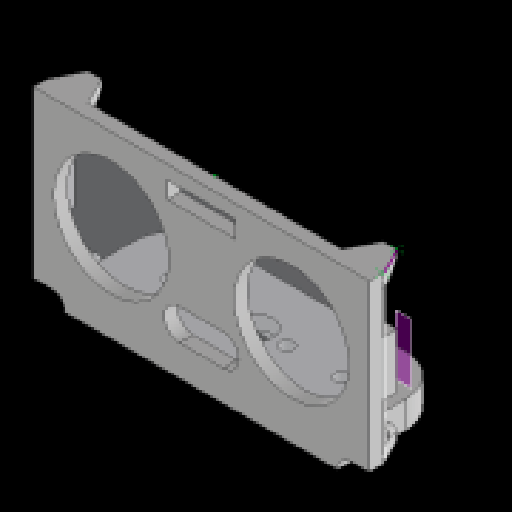
# Autodesk Inventor part: ultrasomicHolder
Saved by Autodesk Inventor 2024.3 (Build 283343010, 343A)
## iProperties
Created: 2025-05-13
Part Number: ultrasomicHolder
Material: Generic
Document SubType Name: Modeling
Designer: Oleg Kelner
Density: 1 g/cm^3
Appearance: Default
Author: Oleg Kelner
Autodesk Inventor part; units mm, degrees
ref_plane "YZ Plane" through (0, 0, 0) normal (1, 0, 0) x (0, 1, 0)
ref_plane "XZ Plane" through (0, 0, 0) normal (0, 1, 0) x (-1, 0, 0)
ref_plane "XY Plane" through (0, 0, 0) normal (0, 0, 1) x (1, 0, 0)
ref_plane "Work Plane1" through (0, 0, 0) normal (0, 0, 1) x (1, 0, 0)
sketch "Sketch1" plane through (0, 0, 0) normal (0, 0, 1) x (1, 0, 0)
  line L0 (-22.65, -10.15) -> (22.65, -10.15) construction
  line L1 (22.65, -10.15) -> (22.65, 10.15) construction
  line L2 (22.65, 10.15) -> (-22.65, 10.15) construction
  line L3 (-22.65, 10.15) -> (-22.65, -10.15) construction
  line L4 (3.2, -5.55) -> (-3.2, -5.55) construction
  arc A0 (3.2, -9.15) -> (3.2, -5.55) centre (3.2, -7.35) ccw construction
  line L5 (-3.2, -9.15) -> (3.2, -9.15) construction
  arc A1 (-3.2, -5.55) -> (-3.2, -9.15) centre (-3.2, -7.35) ccw construction
  circle A2 centre (-13.25, 0) radius 7.95 construction
  circle A3 centre (13.25, 0) radius 7.95 construction
  circle A4 centre (-21.75, -9.25) radius 0.75 construction
  circle A5 centre (-21.75, 9.25) radius 0.75 construction
  circle A6 centre (21.75, 9.25) radius 0.75 construction
  circle A7 centre (21.75, -9.25) radius 0.75 construction
  line L6 (-24.65, 12.15) -> (24.65, 12.15)
  line L7 (24.65, 12.15) -> (24.65, -12.15)
  line L8 (24.65, -12.15) -> (-24.65, -12.15)
  line L9 (-24.65, -12.15) -> (-24.65, 12.15)
  circle A8 centre (-13.25, 0) radius 8.45
  circle A9 centre (13.25, 0) radius 8.45
  line L10 (-3.2, -5.05) -> (3.2, -5.05)
  arc A10 (3.2, -9.65) -> (3.2, -5.05) centre (3.2, -7.35) ccw
  line L11 (3.2, -9.65) -> (-3.2, -9.65)
  arc A11 (-3.2, -5.05) -> (-3.2, -9.65) centre (-3.2, -7.35) ccw
  point P0 (0, 0)
  dimension "d0" = 2
  dimension "d1" = 0.5
  dimension "d2" = 0.5
  dimension "d3" = 0.5
  constraints: 12 end point, 4 centre point, 4 point on circle, 6 other
  measures "d0" distance between parallel lines of L2 L6
  measures "d1" radial gap between concentric circles of A2 A8
  measures "d2" radial gap between concentric circles of A3 A9
  measures "d3" distance between parallel lines of L4 L10
extrude "Extrusion1" add sketch "Sketch1" along normal blind 2
sketch "Sketch5" plane through (0, 0, 0) normal (0, 0, -1) x (-1, 0, 0)
  line L0 (24.65, -12.15) -> (-24.65, -12.15) construction
  line L1 (24.65, 12.15) -> (24.65, -12.15) construction
  line L2 (-24.65, 12.15) -> (24.65, 12.15) construction
  line L3 (-24.65, -12.15) -> (-24.65, 12.15) construction
  circle A0 centre (13.25, 0) radius 8.45 construction
  circle A1 centre (-13.25, 0) radius 8.45 construction
  line L4 (-3.2, -9.65) -> (3.2, -9.65) construction
  arc A2 (-3.2, -5.05) -> (-3.2, -9.65) centre (-3.2, -7.35) ccw construction
  line L5 (3.2, -5.05) -> (-3.2, -5.05) construction
  arc A3 (3.2, -9.65) -> (3.2, -5.05) centre (3.2, -7.35) ccw construction
  line L6 (22.65, -10.15) -> (-22.65, -10.15) construction
  line L7 (-22.65, -10.15) -> (-22.65, 10.15) construction
  line L8 (-22.65, 10.15) -> (22.65, 10.15) construction
  line L9 (22.65, 10.15) -> (22.65, -10.15) construction
  line L10 (-3.2, -5.55) -> (3.2, -5.55) construction
  arc A4 (-3.2, -5.55) -> (-3.2, -9.15) centre (-3.2, -7.35) ccw construction
  line L11 (3.2, -9.15) -> (-3.2, -9.15) construction
  arc A5 (3.2, -9.15) -> (3.2, -5.55) centre (3.2, -7.35) ccw construction
  circle A6 centre (13.25, 0) radius 7.95 construction
  circle A7 centre (-13.25, 0) radius 7.95 construction
  circle A8 centre (21.75, -9.25) radius 0.75 construction
  circle A9 centre (21.75, 9.25) radius 0.75 construction
  circle A10 centre (-21.75, 9.25) radius 0.75 construction
  circle A11 centre (-21.75, -9.25) radius 0.75 construction
  line L12 (-24.65, 4) -> (-24.65, -4)
  line L13 (-24.65, -4) -> (-22.65, -4)
  line L14 (-22.65, -4) -> (-22.65, 4)
  line L15 (-22.65, 4) -> (-24.65, 4)
  line L16 (0, 12.15) -> (0, -12.15)
  line L17 (-24.65, 12.15) -> (-18.65, 12.15)
  line L18 (-18.65, 12.15) -> (-18.65, 10.15)
  line L19 (-18.65, 10.15) -> (-24.65, 10.15)
  line L20 (-24.65, 10.15) -> (-24.65, 12.15)
  line L21 (-24.65, 0) -> (24.65, 0)
  line L22 (24.65, -12.15) -> (24.65, 12.15) construction
  line L23 (22.65, -10.15) -> (22.65, 10.15) construction
  line L24 (24.65, 4) -> (24.65, -4)
  line L25 (24.65, -4) -> (22.65, -4)
  line L26 (22.65, -4) -> (22.65, 4)
  line L27 (22.65, 4) -> (24.65, 4)
  point P0 (0, 0)
  point P1 (-21.65, 10.15)
  dimension "d14" = 8
  dimension "d15" = 6
  constraints: 32 end point, 8 point on line, 6 midpoint, 4 parallel, 4 symmetric about line, 2 perpendicular
  measures "d14" distance between parallel lines of L13 L15
  measures "d15" distance of L2.start L17.end
extrude "Extrusion5" add sketch "Sketch5" along normal blind 2 contours L15 L14 L21 L12 | L21 L14 L13 L12 | L26 L27 L24 L21 | L21 L24 L25 L26
ref_plane "Work Plane2" through (0, 0, -4) normal (0, 0, -1) x (-1, 0, 0)
sketch "Sketch6" plane through (0, 0, -4) normal (0, 0, -1) x (-1, 0, 0)
  line L0 (-24.65, 12.15) -> (24.65, 12.15) projected
  line L1 (-22.65, 10.15) -> (-22.65, 12.15)
  line L2 (-22.65, 12.15) -> (-20.65, 12.15)
  line L3 (-20.65, 12.15) -> (-20.65, 10.15)
  line L4 (-20.65, 10.15) -> (-22.65, 10.15)
  line L5 (-24.65, 0) -> (24.65, 0) projected
  point P0 (-22.65, -10.15)
  point P1 (22.65, 10.15)
  point P2 (22.65, -10.15)
  dimension "d19" = 2
  constraints: 8 end point, 2 parallel, 1 perpendicular, 1 point on line, 1 symmetric about line, 1 vertical, 1 other
  measures "d19" distance of L1.end L2.end
sketch "Sketch7" plane through (24.65, 12.15, 2) normal (0, 1, 0) x (0, 0, -1)
  line L0 (2, 0) -> (6, 2)
  point P0 (2, 24.65)
  constraints: 2 end point
loft "Loft1" add profiles "Sketch5", "Sketch6" contours L17 L18 L19 L20 / all
sketch "Sketch8" plane through (18.65, 10.15, 0) normal (0, -1, 0) x (1, 0, 0)
  line L0 (0, 0) -> (6, 0) projected
  line L1 (0, 0) -> (2, -4) projected
  line L2 (2, -4) -> (4, -4) projected
  line L3 (6, 0) -> (4, -4) projected
  line L4 (-41.3, -1.65) -> (4, -1.65) projected
  line L5 (4, -1.65) -> (5.175, -1.65)
  point P0 (-18.65, 0)
  point P1 (0.825, -1.65)
  constraints: 2 end point, 1 horizontal, 1 point on line
extrude "Extrusion6" add sketch "Sketch8" along normal blind 1 contours L4 L5 L3 L2 L1
pattern_linear "Rectangular Pattern1" count 2 spacing 43.3 along (-1, 0, 0) of "Loft1", "Extrusion6"
mirror "Mirror1" about plane through (0, 0, 0) normal (0, 1, 0) of "Loft1", "Extrusion6", "Rectangular Pattern1"
sketch "Sketch9" plane through (24.65, -12.15, 2) normal (1, 0, 0) x (0, 0, -1)
  line L0 (2, 0) -> (2, 2) projected
  line L1 (2, 8.15) -> (4, 8.15) projected
  line L2 (4, 16.15) -> (4, 8.15) projected
  line L3 (2, 16.15) -> (4, 16.15) projected
  line L4 (2, 16.15) -> (2, 22.3) projected
  line L5 (2, 22.3) -> (2, 24.3) projected
  line L6 (2, 24.3) -> (0, 24.3) projected
  line L7 (0, 0) -> (0, 24.3) projected
  line L8 (2, 0) -> (0, 0) projected
  line L9 (2, 22.3) -> (2, 24.3) projected
  line L10 (2, 22.3) -> (3.65, 22.3) projected
  line L11 (3.65, 22.3) -> (3.65, 21.3) projected
  line L12 (6, 21.3) -> (3.65, 21.3) projected
  line L13 (6, 21.3) -> (6, 24.3) projected
  line L14 (2, 24.3) -> (6, 24.3) projected
  line L15 (2, 2) -> (2, 8.15) projected
  line L16 (2, 0) -> (2, 2) projected
  line L17 (2, 0) -> (6, 0) projected
  line L18 (6, 3) -> (6, 0) projected
  line L19 (6, 3) -> (3.65, 3) projected
  line L20 (3.65, 2) -> (3.65, 3) projected
  line L21 (2, 2) -> (3.65, 2) projected
  line L22 (6, 2) -> (3.9, 3)
  line L23 (3.65, 2) -> (3.9, 2)
  line L24 (3.9, 2) -> (3.9, 3)
  line L25 (3.65, 22.3) -> (3.9, 22.3)
  line L26 (3.9, 22.3) -> (3.9, 21.3)
  line L27 (6, 22.3) -> (3.9, 21.3)
  point P0 (2, 12.15)
  dimension "d51" = 0.25
  dimension "d52" = 0.25
  constraints: 12 end point, 5 point on line, 2 horizontal, 2 perpendicular
  measures "d51" distance between parallel lines of L20 L24
  measures "d52" distance between parallel lines of L11 L26
extrude "Extrusion8" cut sketch "Sketch9" against normal through all contours L8 L7 L6 L5 L4 L3 L2 L1 L15 L0 | L0 L21 L23 L24 L22 L18 L17 | L14 L13 L27 L26 L25 L10 L5 keep common part
fillet "Fillet1" radius 1 12 edges at (-21.65, -10.15, -4) (-23.175, -9.65, -2.95) (-20.125, -9.65, -2.95) (21.65, -10.15, -4) (20.125, -9.65, -2.95) (23.175, -9.65, -2.95) (-21.65, 10.15, -4) (-23.175, 9.65, -2.95) (-20.125, 9.65, -2.95) (21.65, 10.15, -4) (20.125, 9.65, -2.95) (23.175, 9.65, -2.95)
sketch "Sketch10" plane through (-24.65, -12.15, 2) normal (0, -1, 0) x (1, 0, 0)
  line L0 (37.15, -8) -> (12.15, -8) construction
  line L1 (6, -2) -> (43.3, -2) projected
  line L2 (37.15, -4.4) -> (12.15, -4.4)
  line L3 (12.15, -11.6) -> (37.15, -11.6)
  arc A0 (37.15, -11.6) -> (37.15, -4.4) centre (37.15, -8) ccw
  arc A1 (12.15, -4.4) -> (12.15, -11.6) centre (12.15, -8) ccw
  line L4 (44.65, -16) -> (44.65, 0)
  line L5 (44.65, 0) -> (4.65, 0)
  line L6 (4.65, 0) -> (4.65, -16)
  line L7 (4.65, -16) -> (44.65, -16)
  line L8 (44.65, -16) -> (4.65, 0) construction
  line L9 (44.65, 0) -> (4.65, -16) construction
  line L10 (0, 0) -> (49.3, 0) projected
  point P0 (24.65, -8)
  point P1 (8.55, -8)
  point P2 (40.75, -8)
  point P3 (24.65, 0)
  dimension "d49" = 6
  dimension "d34" = 12.5
  dimension "d35" = 7.2
  dimension "d36" = 32.2
  dimension "d37" = 40
  constraints: 16 end point, 6 point on circle, 4 midpoint, 4 tangent, 3 parallel, 2 centre point, 1 perpendicular, 1 vertical, 7 other
  measures "d34" distance of point (24.65, -8) A1.centre
  measures "d35" diameter of A1
  measures "d36" distance of point (8.55, -8) point (40.75, -8)
  measures "d37" distance between parallel lines of L6 L4
extrude "Extrusion9" add sketch "Sketch10" against normal blind 2 contours A0 L3 A1 L2 | L7 L6 L5 L4
sketch "Sketch11" plane through (-24.65, -12.15, 2) normal (0, -1, 0) x (1, 0, 0)
  arc A0 (37.15, -11.6) -> (37.15, -4.4) centre (37.15, -8) ccw projected
  line L0 (12.15, -11.6) -> (37.15, -11.6) projected
  arc A1 (12.15, -4.4) -> (12.15, -11.6) centre (12.15, -8) ccw projected
  line L1 (37.15, -4.4) -> (12.15, -4.4) projected
  line L2 (44.65, -16) -> (44.65, 0) projected
  line L3 (4.65, 0) -> (4.65, -16) projected
  line L4 (0, 0) -> (49.3, 0) projected
  line L5 (4.65, -16) -> (44.65, -16) projected
  point P0 (24.65, -2)
  constraints: 1 other
extrude "Extrusion10" add sketch "Sketch11" along normal blind 2
fillet "Fillet2" radius 2 2 edges at (20, -12.15, -0.35) (-20, -12.15, -0.35)
sketch "Sketch12" plane through (-12.5, -12.15, -2.4) normal (0, -1, 0) x (1, 0, 0)
  arc A0 (25, -7.2) -> (25, 0) centre (25, -3.6) ccw projected
  line L0 (25, 0) -> (0, 0) projected
  arc A1 (0, 0) -> (0, -7.2) centre (0, -3.6) ccw projected
  line L1 (0, -7.2) -> (25, -7.2) projected
  line L2 (25, -3.6) -> (0, -3.6) construction
  circle A2 centre (25, -3.6) radius 1
  circle A3 centre (17, -3.6) radius 1
  line L3 (12.5, -7.2) -> (12.5, 2.4) construction
  circle A4 centre (0, -3.6) radius 1
  circle A5 centre (8, -3.6) radius 1
  circle A6 centre (12.5, -3.6) radius 2.5
  point P0 (0, -3.6)
  dimension "d43" = 2
  dimension "d44" = 12.5
  dimension "d45" = 2
  dimension "d46" = 4.5
  dimension "d55" = 5
  constraints: 5 centre point, 4 end point, 3 symmetric about line, 2 midpoint, 2 point on line, 1 coincident, 1 horizontal, 1 perpendicular, 2 other
  measures "d43" diameter of A2
  measures "d44" distance of A2.centre point (12.5, -3.6)
  measures "d45" diameter of A3
  measures "d46" distance of point (12.5, -3.6) A3.centre
  measures "d55" diameter of A6
extrude "Extrusion11" cut sketch "Sketch12" against normal blind 2 contours A2 | A3 | A4 | A5 | A6
fillet "Fillet3" radius 6 2 edges at (20, -12.15, -14) (-20, -12.15, -14)
sketch "Sketch13" plane through (0, 0, 2) normal (0, 0, 1) x (1, 0, 0)
  line L0 (5, 10.15) -> (5, 7.65) projected
  line L1 (5, 7.65) -> (-5, 7.65) projected
  line L2 (-5, 7.65) -> (-5, 10.15) projected
  line L3 (-5, 10.15) -> (5, 10.15) projected
  line L4 (-4.05, 9.2) -> (-3.45, 9.2) projected
  line L5 (-4.05, 8.6) -> (-4.05, 9.2) projected
  line L6 (-3.45, 8.6) -> (-4.05, 8.6) projected
  line L7 (-3.45, 9.2) -> (-3.45, 8.6) projected
  line L8 (-1.55, 9.2) -> (-0.95, 9.2) projected
  line L9 (-1.55, 8.6) -> (-1.55, 9.2) projected
  line L10 (-0.95, 8.6) -> (-1.55, 8.6) projected
  line L11 (-0.95, 9.2) -> (-0.95, 8.6) projected
  line L12 (0.95, 9.2) -> (1.55, 9.2) projected
  line L13 (0.95, 8.6) -> (0.95, 9.2) projected
  line L14 (1.55, 8.6) -> (0.95, 8.6) projected
  line L15 (1.55, 9.2) -> (1.55, 8.6) projected
  line L16 (3.45, 9.2) -> (4.05, 9.2) projected
  line L17 (3.45, 8.6) -> (3.45, 9.2) projected
  line L18 (4.05, 8.6) -> (3.45, 8.6) projected
  line L19 (4.05, 9.2) -> (4.05, 8.6) projected
  point P0 (0, 0)
extrude "Extrusion12" cut sketch "Sketch13" against normal through all contours L0 L1 L2 L3 | L4 L7 L6 L5 | L8 L11 L10 L9 | L12 L15 L14 L13 | L16 L19 L18 L17
body "Solid1"
